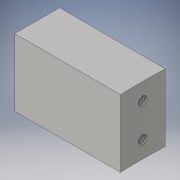
# Autodesk Inventor part: mountingStub
Saved by Autodesk Inventor 2016 (Build 200138000, 138)
## iProperties
Created: 2015-12-10
Part Number: mountingStub
Material: Generic
Document SubType Name: Modeling
Designer: Dave
Density: 1 g/cm^3
Appearance: Default
Author: Dave
Autodesk Inventor part; units mm, degrees
ref_plane "YZ Plane" through (0, 0, 0) normal (1, 0, 0) x (0, 1, 0)
ref_plane "XZ Plane" through (0, 0, 0) normal (0, 1, 0) x (-1, 0, 0)
ref_plane "XY Plane" through (0, 0, 0) normal (0, 0, 1) x (1, 0, 0)
sketch "Sketch1" plane through (0, 0, 0) normal (0, 1, 0) x (-1, 0, 0)
  line L0 (0, 0) -> (63.5, 0)
  line L1 (63.5, 0) -> (63.5, -25.4)
  line L2 (63.5, -25.4) -> (0, -25.4)
  line L3 (0, -25.4) -> (0, 0)
  dimension "d0" = 25.4
  dimension "d1" = 63.5
  constraints: 8 end point, 2 parallel, 1 horizontal, 1 perpendicular
  measures "d0" distance of L2.end L0.start
  measures "d1" distance of L0.start L0.end
extrude "Extrusion1" add sketch "Sketch1" along normal blind 38.1
sketch "Sketch3" plane through (0, 0, 0) normal (1, 0, 0) x (0, 0, -1)
  circle A0 centre (12.7, 28.575) radius 2.581
  line L0 (0, 38.1) -> (25.4, 38.1) projected
  circle A1 centre (12.7, 9.525) radius 2.3807
  point P0 (0, 0)
  dimension "d6" = 9.525
  dimension "d7" = 19.05
  constraints: 2 centre point
  measures "d6" distance from line of A0.centre L0
  measures "d7" distance of A1.centre A0.centre
hole "Hole1" at (0, 28.575, -12.7) at (0, 9.525, -12.7) direction (-1, 0, 0) diameter 4.9784 end through all thread size "1/4-20 UNC" class "2B" standard "ANSI Unified Screw Threads"
sketch "Sketch4" plane through (0, 38.1, 0) normal (0, 1, 0) x (1, 0, 0)
  line L0 (0, 0) -> (0, 25.4) projected
  line L1 (0, 12.7) -> (326.39, 12.7) construction
  circle A0 centre (326.39, 12.7) radius 330.2
  dimension "d15" = 326.39
  dimension "d16" = 660.4
  constraints: 2 end point, 1 centre point, 1 coincident, 1 horizontal, 1 midpoint
  measures "d15" distance of L1.start L1.end
  measures "d16" diameter of A0
extrude "Extrusion2" cut sketch "Sketch4" against normal blind 50.8
body "Solid1"
